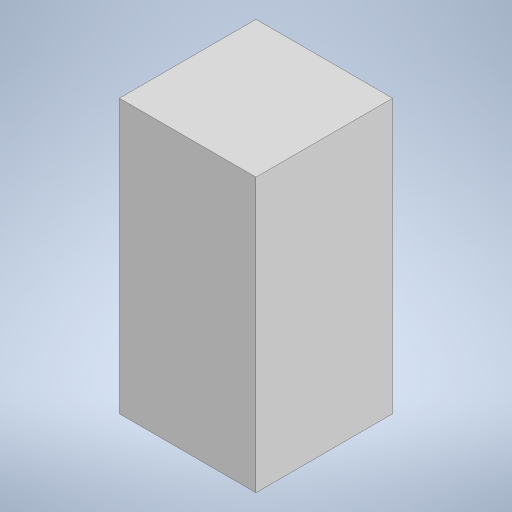
# Autodesk Inventor part: stand
Saved by Autodesk Inventor 2023 (Build 270158000, 158)
## iProperties
Created: 2022-06-19
Part Number: stand
Material: Generic
Document SubType Name: Modeling
Designer: ADITYA CHINAGUDI
Density: 1 g/cm^3
Appearance: Default
Author: ADITYA CHINAGUDI
Autodesk Inventor part; units mm, degrees
ref_plane "YZ Plane" through (0, 0, 0) normal (1, 0, 0) x (0, 1, 0)
ref_plane "XZ Plane" through (0, 0, 0) normal (0, 1, 0) x (-1, 0, 0)
ref_plane "XY Plane" through (0, 0, 0) normal (0, 0, 1) x (1, 0, 0)
sketch "Sketch1" plane through (0, 0, 0) normal (0, 0, 1) x (1, 0, 0)
  line L0 (-8.3656, 8.322) -> (21.6344, 8.322)
  line L1 (21.6344, 8.322) -> (21.6344, -51.678)
  line L2 (21.6344, -51.678) -> (-8.3656, -51.678)
  line L3 (-8.3656, -51.678) -> (-8.3656, 8.322)
  point P0 (0, 0)
  dimension "d0" = 30
  dimension "d1" = 60
  constraints: 8 end point, 2 parallel, 1 horizontal, 1 perpendicular
  measures "d0" distance of L1.end L2.end
  measures "d1" distance of L0.end L1.end
extrude "Extrusion1" add sketch "Sketch1" along normal blind 30
body "Solid1"
